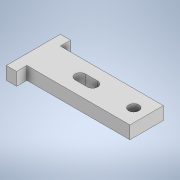
# Autodesk Inventor part: motor_fastening
Saved by Autodesk Inventor 2022 (Build 260153000, 153)
## iProperties
Created: 2022-02-09
Part Number: motor_fastening
Material: Generic
Document SubType Name: Modeling
Designer: Iñigo
Density: 1 g/cm^3
Appearance: Default
Author: Iñigo
Autodesk Inventor part; units mm, degrees
ref_plane "YZ Plane" through (0, 0, 0) normal (1, 0, 0) x (0, 1, 0)
ref_plane "XZ Plane" through (0, 0, 0) normal (0, 1, 0) x (-1, 0, 0)
ref_plane "XY Plane" through (0, 0, 0) normal (0, 0, 1) x (1, 0, 0)
sketch "Sketch1" plane through (0, 0, 0) normal (0, 1, 0) x (-1, 0, 0)
  line L0 (10, -6.5) -> (-30, -6.5)
  line L1 (10, -10.5) -> (14, -10.5)
  line L2 (14, -10.5) -> (14, 0)
  line L3 (10, -6.5) -> (10, -10.5)
  line L4 (-30, 0) -> (-30, -6.5)
  line L5 (10, 6.5) -> (-30, 6.5)
  line L6 (10, 10.5) -> (14, 10.5)
  line L7 (14, 10.5) -> (14, 0)
  line L8 (10, 6.5) -> (10, 10.5)
  line L9 (-30, 0) -> (-30, 6.5)
  point P0 (0, 0)
  dimension "d0" = 40
  dimension "d5" = 4
  dimension "d15" = 13
  constraints: 20 end point, 1 parallel
  measures "d0" distance of L0.start L0.end
  measures "d5" distance between parallel lines of L0 L1
  measures "d15" distance between parallel lines of L5 L0
extrude "Extrusion1" add sketch "Sketch1" along normal blind 5
sketch "Sketch2" plane through (0, 5, 0) normal (0, 1, 0) x (1, 0, 0)
  circle A0 centre (25, 0) radius 2
  arc A1 (9, -2) -> (9, 2) centre (9, 0) ccw
  arc A2 (4.1943, 2) -> (4.1943, -2) centre (4.1943, 0) ccw
  line L0 (9, -2) -> (4.1943, -2)
  line L1 (4.1943, 2) -> (9, 2)
  point P0 (0, 0)
  dimension "d8" = 4
  dimension "d10" = 4
  dimension "d11" = 12
  dimension "d12" = 4
  constraints: 4 end point, 4 point on circle, 3 centre point, 3 tangent
  measures "d8" diameter of A0
  measures "d10" diameter of A1
  measures "d12" diameter of A2
extrude "Extrusion2" cut sketch "Sketch2" against normal blind 7.75
body "Solid1"
